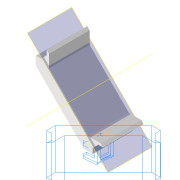
# Autodesk Inventor part: 20_Cube_Insert_Mirror_Holder_wLogo_Astromedia_30x40x1_v3
Saved by Autodesk Inventor 2022 (Build 260153000, 153)
## iProperties
Created: 2019-07-22
Part Number: 20_Cube_Insert_Mirror_Holder_wLogo_Astromedia_30x40x1_v3
Material: Generic
Document SubType Name: Modeling
Designer: diederichbenedict
Density: 1 g/cm^3
Appearance: Default
Mass: 16.3755 g
Surface Area: 59.344 cm^2
Volume: 16.3755 cm^3
Catalog Web Link: isPrinted
Vendor: openUC2
Author: diederichbenedict
Autodesk Inventor part; units mm, degrees
ref_plane "YZ Plane" through (0, 0, 0) normal (1, 0, 0) x (0, 1, 0)
ref_plane "XZ Plane" through (0, 0, 0) normal (0, 1, 0) x (-1, 0, 0)
sketch "Sketch1" plane through (0, 0, 0) normal (0, 0, 1) x (1, 0, 0)
  line L0 (21.1431, -16.9027) -> (16.9281, -21.1177)
  line L1 (-21.2613, 16.9973) -> (-17.0227, 21.2358)
  line L2 (-17.0227, 21.2358) -> (16.9281, -21.1177) construction
  line L3 (21.1431, -16.9027) -> (-21.2613, 16.9973) construction
  line L4 (-17.0227, 21.2358) -> (36.8231, 21.2358) construction
  line L5 (16.9281, -21.1177) -> (16.9281, -25.0027)
  line L6 (-17.0227, 21.2358) -> (-17.0227, 24.8927)
  line L7 (21.1431, -16.9027) -> (24.7727, -16.9027)
  line L8 (24.7727, -16.9027) -> (-17.0227, 24.8927)
  line L9 (-25.0027, 16.9973) -> (-25.0027, 10.6306)
  line L10 (16.9281, -25.0027) -> (10.6306, -25.0027)
  line L11 (-25.0027, 10.6306) -> (10.6306, -25.0027)
  line L12 (-25.0027, 16.9973) -> (-7.0741, 16.9973) construction
  line L13 (-17.1227, 21.2773) -> (-21.3027, 17.0973)
  line L14 (16.8927, -21.1827) -> (21.0727, -17.0027)
  line L15 (24.7727, -17.0027) -> (21.1414, -17.0027)
  line L16 (22.7727, -25.0027) -> (-23.0273, -25.0027)
  line L17 (16.8927, -25.0027) -> (16.8927, -21.2526)
  line L18 (-17.1227, 25.0973) -> (-17.1227, 21.3471)
  line L19 (-25.0027, 17.0973) -> (-21.3714, 17.0973)
  line L20 (-21.2613, 16.9973) -> (-25.0027, 16.9973)
  point P0 (0, 0)
  point P1 (16.8927, -21.2526)
extrude "Extrusion1" add sketch "Sketch1" along normal blind 30
ref_plane "Work Plane1" through (16.9, -16.9, -8) normal (-0.7071068, -0.7071068, 0) x (0, 0, 1)
sketch "Sketch7" plane through (0, 0, 30) normal (0, 0, 1) x (1, 0, 0)
  line L0 (21.1431, -16.9027) -> (24.7727, -16.9027) projected
  line L1 (24.7727, -16.9027) -> (-17.0227, 24.8927) projected
  line L2 (-17.0227, 24.8927) -> (-17.0227, 21.2358) projected
  line L3 (-17.0227, 21.2358) -> (-21.2613, 16.9973) projected
  line L4 (-21.2613, 16.9973) -> (-25.0027, 16.9973) projected
  line L5 (-25.0027, 16.9973) -> (-25.0027, 10.6306) projected
  line L6 (-25.0027, 10.6306) -> (10.6306, -25.0027) projected
  line L7 (10.6306, -25.0027) -> (16.9281, -25.0027) projected
  line L8 (16.9281, -25.0027) -> (16.9281, -21.1177) projected
  line L9 (16.9281, -21.1177) -> (21.1431, -16.9027) projected
  line L10 (3.875, 3.995) -> (-7.1861, -7.1861)
  line L11 (-25.0027, 10.6306) -> (10.6306, -25.0027) projected
  line L12 (23.0128, -5.8586) -> (13.7286, -15.1428)
  line L13 (13.7286, -15.1428) -> (-15.2628, 13.8486)
  line L14 (-15.2628, 13.8486) -> (-5.9786, 23.1328)
  line L15 (-5.9786, 23.1328) -> (23.0128, -5.8586)
  line L16 (23.0128, -5.8586) -> (-15.2628, 13.8486) construction
  line L17 (13.7286, -15.1428) -> (-5.9786, 23.1328) construction
  line L18 (-15.2628, 13.8486) -> (-15.2628, 23.1328)
  line L19 (24.7727, -16.9027) -> (-17.0227, 24.8927) projected
  line L20 (13.7286, -15.1428) -> (23.0128, -15.1428)
  point P0 (0, 0)
  dimension "d28" = 41
  dimension "d29" = 1
  dimension "d74" = 0
  constraints: 18 end point, 4 midpoint, 2 parallel, 2 perpendicular, 2 point on line, 1 vertical
  measures "d28" distance of L12.end L13.end
  measures "d29" distance from line of L13 point (0, 0)
  measures "d74" angle of L1 L15
extrude "Extrusion7" cut sketch "Sketch7" against normal through all contours L20 L12 L1 | L12 L13 L10 L1 | L1 L14 L15 L12 | L10 L13 L14 L1 | L14 L18 L1
sketch "Sketch10" plane through (10.6306, -25.0027, 30) normal (-0.7071068, -0.7071068, 0) x (-0.7071068, 0.7071068, 0)
  line L0 (1.6838, 16.5215) -> (7.0744, 19.4702) construction
  line L1 (7.0744, 19.4702) -> (7.0744, 10.5304) construction
  line L2 (7.0744, 10.5304) -> (1.6838, 10.5304) construction
  line L3 (1.6838, 10.5304) -> (1.6838, 6.839) construction
  line L4 (1.6838, 6.839) -> (6.7206, 6.839) construction
  line L5 (6.7206, 6.839) -> (6.7206, 1.2092) construction
  line L6 (6.7206, 1.2092) -> (1.6838, 1.2092) construction
  line L7 (1.6838, 1.2092) -> (1.6838, -3.423) construction
  line L8 (1.6838, -3.423) -> (55.1934, -3.423) construction
  line L9 (1.6838, 30.377) -> (1.6838, 26.2152) construction
  line L10 (1.6838, 26.2152) -> (7.1181, 26.2152) construction
  line L11 (7.1181, 26.2152) -> (7.1181, 20.0634) construction
  line L12 (7.1181, 20.0634) -> (1.6838, 20.0634) construction
  line L13 (1.6838, 20.0634) -> (1.6838, 16.5215) construction
  line L14 (7.0744, 15.0003) -> (55.1934, 14.9149) construction
  line L15 (1.6838, 30.377) -> (36.6838, 30.377) construction
  line L16 (36.6838, -3.423) -> (1.6838, -3.423) construction
  line L17 (19.8996, 21.1501) -> (19.8996, 11.1501)
  line L18 (19.8996, 11.1501) -> (28.5599, 6.1501)
  line L19 (19.8996, 21.1501) -> (21.3996, 20.2841)
  line L20 (21.3996, 20.2841) -> (21.3996, 12.0161)
  line L21 (21.3996, 12.0161) -> (27.0599, 8.7482)
  line L22 (27.0599, 8.7482) -> (27.0599, 17.0161)
  line L23 (27.0599, 17.0161) -> (28.5599, 16.1501)
  line L24 (28.5599, 16.1501) -> (28.5599, 6.1501)
  line L25 (50.3931, 0) -> (0, 0) construction
  line L26 (50.3931, 30) -> (50.3931, 0) construction
  line L27 (50.3931, 15) -> (0, 15) construction
  line L28 (0, 30) -> (0, 0) construction
  point P0 (25.1966, 30)
  point P1 (25.1966, 15)
  dimension "d40" = 1.5
  dimension "d41" = 1.5
  dimension "d42" = 1.5
  dimension "d43" = 10
  dimension "d44" = 10
  dimension "d75" = 8.268
  dimension "d76" = 120
  constraints: 52 end point, 4 midpoint, 4 parallel, 2 collinear, 1 vertical
  measures "d40" distance between parallel lines of L20 L17
  measures "d41" distance between parallel lines of L24 L22
  measures "d42" distance between parallel lines of L18 L21
  measures "d43" distance of L17.start L17.end
  measures "d44" distance of L17.end L18.end
  measures "d75" distance of L21.end L22.end
  measures "d76" angle of L21 L22
emboss "Emboss1" sketch "Sketch10" operation cut depth 1 direction (0.7071068, 0.7071068, 0)
sketch "Sketch11" plane through (10.6306, -25.0027, 30) normal (-0.7071068, -0.7071068, 0) x (-0.7071068, 0.7071068, 0)
  line L0 (21.3996, 12.0161) -> (27.0599, 8.7482) construction
  line L1 (27.0599, 8.7482) -> (27.0599, 17.0161) construction
  line L2 (27.0599, 17.0161) -> (28.5599, 16.1501) construction
  line L3 (28.5599, 16.1501) -> (28.5599, 6.1501) construction
  line L4 (28.5599, 6.1501) -> (19.8996, 11.1501) construction
  line L5 (19.8996, 11.1501) -> (19.8996, 21.1501) construction
  line L6 (19.8996, 21.1501) -> (21.3996, 20.2841) construction
  line L7 (21.3996, 20.2841) -> (21.3996, 12.0161) construction
  line L8 (50.3931, 30) -> (0, 30) construction
  line L9 (0, 30) -> (0, 0) construction
  line L10 (50.3931, 0) -> (0, 0) construction
  line L11 (50.3931, 30) -> (50.3931, 0) construction
  line L12 (9.2379, 27.3057) -> (21.3996, 20.2841) construction
  line L13 (21.3996, 20.2841) -> (21.3996, 12.0161) construction
  line L14 (21.3996, 12.0161) -> (27.0599, 8.7482) construction
  line L15 (27.0599, 8.7482) -> (27.0599, 7.4216) construction
  line L16 (27.0599, 7.4216) -> (17.8982, 13.0177) construction
  line L17 (17.8982, 13.0177) -> (17.8982, 3.0177) construction
  line L18 (17.8982, 3.0177) -> (9.2379, 8.0177) construction
  line L19 (9.2379, 8.0177) -> (9.2379, 27.3057) construction
  line L20 (15.5651, 18.4016) -> (15.5, -16.9) construction
  line L21 (15.5651, 18.4016) -> (-17.5, 16.9) construction
  line L22 (-17.5, 16.9) -> (-17.5, 12.7382) construction
  line L23 (-17.5, 12.7382) -> (-12.0658, 12.7382) construction
  line L24 (-12.0658, 12.7382) -> (-12.0658, 6.5864) construction
  line L25 (-12.0658, 6.5864) -> (-17.5, 6.5864) construction
  line L26 (-17.5, 6.5864) -> (-17.5, 3.0446) construction
  line L27 (-17.5, 3.0446) -> (-12.1095, 3.0446) construction
  line L28 (-12.1095, 3.0446) -> (-12.1095, -2.9465) construction
  line L29 (-12.1095, -2.9465) -> (-17.5, -2.9465) construction
  line L30 (-17.5, -2.9465) -> (-17.5, -6.638) construction
  line L31 (-17.5, -6.638) -> (-12.4632, -6.638) construction
  line L32 (-12.4632, -6.638) -> (-12.4632, -12.2678) construction
  line L33 (-12.4632, -12.2678) -> (-17.5, -12.2678) construction
  line L34 (-17.5, -12.2678) -> (-17.5, -16.9) construction
  line L35 (-17.5, -16.9) -> (15.5, -16.9) construction
  line L36 (-12.1095, 0.049) -> (15.5326, 0.7508) construction
  line L37 (15.5, -16.9) -> (15.5651, 18.4016) construction
  line L38 (1.91, 17.7815) -> (1.91, -16.9) construction
  line L39 (15.5, -16.9) -> (-17.5, -16.9) construction
  line L40 (27.0599, 8.7482) -> (27.0599, 7.4216) construction
  line L41 (21.3996, 20.2841) -> (21.3996, 12.0161)
  line L42 (21.3996, 12.0161) -> (27.0599, 8.7482)
  line L43 (21.3996, 20.2841) -> (21.3996, 12.0161)
  line L44 (21.3996, 12.0161) -> (27.0599, 8.7482)
  line L45 (27.0599, 8.7482) -> (27.0599, 10.4802)
  line L46 (27.0599, 8.7482) -> (27.0599, 7.4216)
  line L47 (27.0599, 10.4802) -> (22.8996, 12.8822)
  line L48 (22.8996, 12.8822) -> (22.8996, 19.4181)
  line L49 (22.8996, 19.4181) -> (27.0599, 21.82)
  line L50 (21.3996, 20.2841) -> (27.0599, 23.552)
  line L51 (27.0599, 23.552) -> (27.0599, 21.82)
  point P0 (25.1966, 30)
  point P1 (20.9754, 14.9785)
  dimension "d47" = 120
  dimension "d48" = 1.5
  dimension "d49" = 1.5
  dimension "d50" = 1.5
  dimension "d77" = 8.268
  dimension "d78" = 4.1602
  dimension "d79" = 5.6602
  dimension "d80" = 120
  dimension "d81" = 120
  constraints: 80 end point, 5 parallel, 3 point on line, 2 collinear, 2 midpoint
  measures "d47" angle of L50 L12
  measures "d48" distance between parallel lines of L13 L48
  measures "d49" distance between parallel lines of L50 L49
  measures "d50" distance between parallel lines of L14 L47
  measures "d77" distance of L0.start L12.end
  measures "d78" distance between parallel lines of L48 L15
  measures "d79" distance between parallel lines of L13 L51
  measures "d80" angle of L48 L47
  measures "d81" angle of L48 L49
emboss "Emboss2" sketch "Sketch11" operation cut depth 1.5 direction (0.7071068, 0.7071068, 0)
sketch "Sketch12" plane through (10.6306, -25.0027, 30) normal (-0.7071068, -0.7071068, 0) x (-0.7071068, 0.7071068, 0)
  line L0 (22.8996, 12.8822) -> (27.0599, 10.4802) construction
  line L1 (27.0599, 10.4802) -> (27.0599, 17.0161) construction
  line L2 (27.0599, 17.0161) -> (28.5599, 16.1501) construction
  line L3 (28.5599, 16.1501) -> (28.5599, 6.1501) construction
  line L4 (28.5599, 6.1501) -> (19.8996, 11.1501) construction
  line L5 (19.8996, 11.1501) -> (19.8996, 21.1501) construction
  line L6 (19.8996, 21.1501) -> (21.3996, 20.2841) construction
  line L7 (21.3996, 20.2841) -> (27.0599, 23.552) construction
  line L8 (27.0599, 23.552) -> (27.0599, 21.82) construction
  line L9 (27.0599, 21.82) -> (22.8996, 19.4181) construction
  line L10 (22.8996, 19.4181) -> (22.8996, 12.8822) construction
  line L11 (50.3931, 30) -> (0, 30) construction
  line L12 (0, 30) -> (0, 0) construction
  line L13 (50.3931, 0) -> (0, 0) construction
  line L14 (50.3931, 30) -> (50.3931, 0) construction
  line L15 (12.7689, 9.4432) -> (16.9291, 7.0413) construction
  line L16 (16.9291, 7.0413) -> (27.0599, 17.0161) construction
  line L17 (27.0599, 17.0161) -> (28.5599, 16.1501) construction
  line L18 (28.5599, 16.1501) -> (28.5599, 6.1501) construction
  line L19 (28.5599, 6.1501) -> (13.0911, 5.9826) construction
  line L20 (13.0911, 5.9826) -> (19.8996, 21.1501) construction
  line L21 (19.8996, 21.1501) -> (21.3996, 20.2841) construction
  line L22 (21.3996, 20.2841) -> (27.0599, 23.552) construction
  line L23 (27.0599, 23.552) -> (27.0599, 21.82) construction
  line L24 (27.0599, 21.82) -> (12.7689, 15.9791) construction
  line L25 (12.7689, 15.9791) -> (12.7689, 9.4432) construction
  line L26 (-17.5, 16.9) -> (-17.5, 12.7382) construction
  line L27 (-17.5, 12.7382) -> (-12.0658, 12.7382) construction
  line L28 (-12.0658, 12.7382) -> (-12.0658, 6.5864) construction
  line L29 (-12.0658, 6.5864) -> (-17.5, 6.5864) construction
  line L30 (-17.5, 6.5864) -> (-17.5, 3.0446) construction
  line L31 (-17.5, 3.0446) -> (-12.1095, 3.0446) construction
  line L32 (-12.1095, 3.0446) -> (-12.1095, -2.9465) construction
  line L33 (-12.1095, -2.9465) -> (-17.5, -2.9465) construction
  line L34 (-17.5, -2.9465) -> (-17.5, -6.638) construction
  line L35 (-17.5, -6.638) -> (-12.4632, -6.638) construction
  line L36 (-12.4632, -6.638) -> (-12.4632, -12.2678) construction
  line L37 (-12.4632, -12.2678) -> (-17.5, -12.2678) construction
  line L38 (-17.5, -12.2678) -> (-17.5, -16.9) construction
  line L39 (-17.5, -16.9) -> (15.5, -16.9) construction
  line L40 (21.3996, 20.2841) -> (27.0599, 23.552)
  line L41 (19.8996, 21.1501) -> (21.3996, 20.2841)
  line L42 (21.3996, 20.2841) -> (27.0599, 23.552)
  line L43 (27.0599, 23.552) -> (27.0599, 21.82)
  line L44 (27.0599, 23.552) -> (27.0599, 21.82)
  line L45 (16.9291, 7.0413) -> (27.0599, 17.0161) construction
  line L46 (19.8996, 21.1501) -> (27.0599, 25.2841)
  line L47 (27.0599, 25.2841) -> (35.7201, 20.2841)
  line L48 (35.7201, 20.2841) -> (35.7201, 18.552)
  line L49 (35.7201, 18.552) -> (30.0599, 15.2841)
  line L50 (30.0599, 15.2841) -> (30.0599, 10.4802)
  line L51 (30.0599, 10.4802) -> (34.2201, 12.8822)
  line L52 (35.7201, 10.2841) -> (35.7201, 10.2841)
  line L53 (35.7201, 10.2841) -> (28.5599, 6.1501)
  line L54 (27.0599, 17.0161) -> (28.5599, 16.1501)
  line L55 (28.5599, 6.1501) -> (28.5599, 16.1501)
  line L56 (28.5599, 16.1501) -> (27.0599, 17.0161)
  line L57 (27.0599, 21.82) -> (27.0599, 23.552)
  line L58 (28.5599, 16.1501) -> (28.5599, 6.1501)
  line L59 (27.0599, 17.0161) -> (31.2201, 19.4181)
  line L60 (31.2201, 19.4181) -> (27.0599, 21.82)
  line L61 (13.0911, 5.9826) -> (28.5599, 6.1501) construction
  line L62 (12.7689, 9.4432) -> (16.9291, 7.0413) construction
  line L63 (12.7689, 9.4432) -> (28.5599, 9.6142) construction
  line L64 (28.5599, 9.6142) -> (29.486, 10.1489) construction
  line L65 (28.5599, 16.1501) -> (35.7201, 20.2841) construction
  line L66 (28.5599, 6.1501) -> (34.2971, 9.4625) construction
  line L67 (31.2201, 19.4181) -> (35.3769, 18.7502) construction
  line L68 (27.0599, 23.552) -> (27.0599, 21.82) construction
  line L69 (35.3769, 18.7502) -> (27.0599, 23.552) construction
  line L70 (35.7201, 10.2841) -> (35.7201, 12.0161)
  line L71 (35.7201, 12.0161) -> (34.2201, 12.8822)
  line L72 (16.3223, 7.4494) -> (20.4826, 5.0475) construction
  line L73 (16.3223, 13.9853) -> (16.3223, 7.4494) construction
  line L74 (20.4826, 16.3872) -> (16.3223, 13.9853) construction
  line L75 (20.4826, 18.1193) -> (20.4826, 16.3872) construction
  line L76 (14.8223, 14.8513) -> (20.4826, 18.1193) construction
  line L77 (14.8223, 15.7065) -> (14.8223, 14.8513) construction
  line L78 (20.4826, 12.5307) -> (14.8223, 15.7065) construction
  line L79 (20.4826, 5.0475) -> (20.4826, 12.5307) construction
  line L80 (20.4826, 12.5307) -> (28.5599, 7.9987) construction
  line L81 (28.5599, 7.9987) -> (33.93, 11.0117) construction
  point P0 (25.1966, 30)
  point P1 (20.9754, 14.9785)
  dimension "d54" = 60
  dimension "d55" = 1.5
  dimension "d57" = 120
  dimension "d58" = 1.5
  dimension "d59" = 120
  dimension "d82" = 3
  dimension "d83" = 3
  dimension "d84" = 3
  dimension "d85" = 1.5
  dimension "d86" = 7.1602
  dimension "d87" = 7.1602
  dimension "d88" = 4.1602
  dimension "d89" = 1.7321
  dimension "d90" = 5.6602
  dimension "d91" = 1.7321
  dimension "d92" = 4.1602
  constraints: 134 end point, 11 parallel, 5 point on line, 4 collinear, 2 vertical, 1 other
  measures "d54" angle of L21 L46
  measures "d55" distance between parallel lines of L50 L18
  measures "d57" angle of L18 L64
  measures "d58" distance between parallel lines of L65 L49
  measures "d59" angle of L70 L71
  measures "d82" distance between parallel lines of L53 L51
  measures "d83" distance between parallel lines of L59 L49
  measures "d84" distance between parallel lines of L47 L60
  measures "d85" distance between parallel lines of L46 L42
  measures "d86" distance between parallel lines of L21 L47
  measures "d87" distance between parallel lines of L47 L17
  measures "d88" distance from line of L50.end L71
  measures "d89" distance of L52.start L70.end
  measures "d90" horizontal distance of L22.end L21.end
  measures "d91" distance of L23.end L22.end
  measures "d92" horizontal distance of L59.end L23.end
extrude "Extrusion9" cut sketch "Sketch12" against normal blind 2
ref_plane "Arbeitsebene4" through (-16.9409, 16.9409, 0) normal (-0.7071068, -0.7071068, 0) x (0, 0, 1)
ref_plane "Arbeitsebene5" through (-2.1793, -2.1793, 0) normal (-0.7071068, 0.7071068, 0) x (-0.7071068, -0.7071068, 0)
equation "\"d3\" = MirrorThickness1"
equation "\"d41\" = d40"
equation "\"d42\" = d40"
equation "\"d44\" = d43"
equation "\"d48\" = d51"
equation "\"d49\" = d51"
equation "\"d50\" = d51"
equation "\"d55\" = d60"
equation "\"d58\" = d60"
equation "\"MirrorThickness1\" = 30"
equation "\"d51\" = 1.5"
equation "\"d60\" = 1.5"
body "Solid1"
